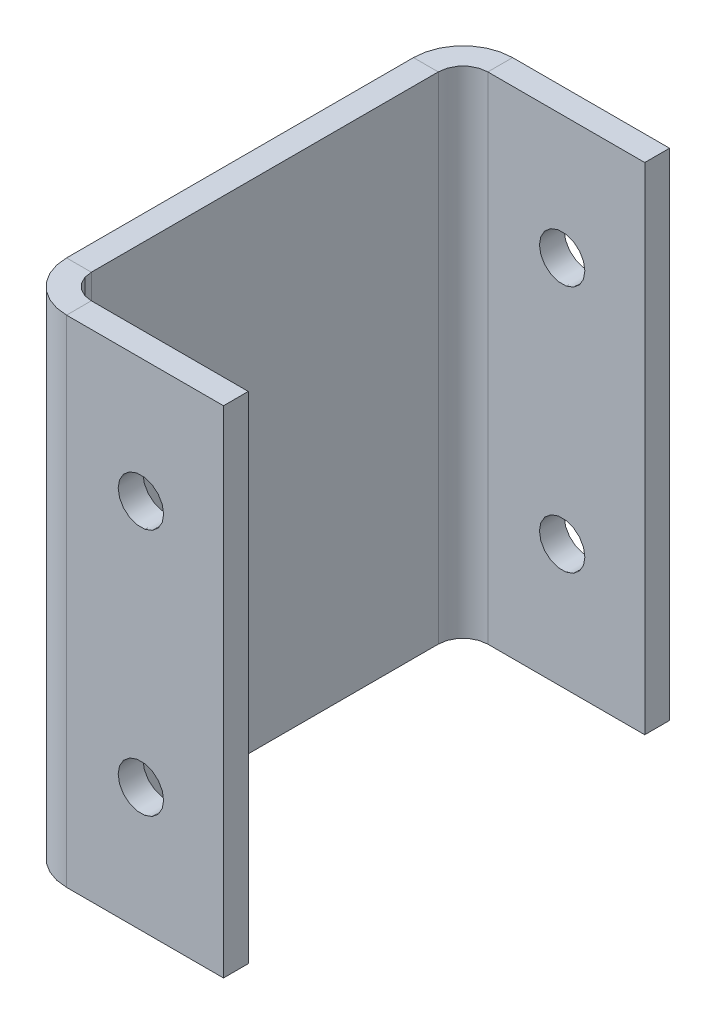
# Autodesk Inventor part: Frontal Sheet Metal Support
Saved by Autodesk Inventor 2019.4 (Build 234330000, 330)
## iProperties
Created: 2020-01-05
Part Number: Frontal Sheet Metal Support
Material: Aluminum 6061
Document SubType Name: Sheet Metal
Designer: Mark
Density: 2.7 g/cm^3
Sheet Metal Rule: Default_mm
Appearance: Aluminum - Flat
Author: Mark
Autodesk Inventor part; units mm, degrees
ref_plane "YZ Plane" through (0, 0, 0) normal (1, 0, 0) x (0, 1, 0)
ref_plane "XZ Plane" through (0, 0, 0) normal (0, 1, 0) x (-1, 0, 0)
ref_plane "XY Plane" through (0, 0, 0) normal (0, 0, 1) x (1, 0, 0)
sketch "Sketch1" plane through (0, 0, 0) normal (1, 0, 0) x (0, 1, 0)
  line L0 (-30, 27) -> (30, 27)
  line L1 (30, 27) -> (30, -27)
  line L2 (30, -27) -> (-30, -27)
  line L3 (-30, -27) -> (-30, 27)
  line L4 (-30, 27) -> (30, -27) construction
  line L5 (30, 27) -> (-30, -27) construction
  point P0 (0, 0)
  dimension "d0" = 60
  dimension "d1" = 54
  measures "d0" distance of L1.end L2.end
  measures "d1" distance of L0.end L1.end
extrude "Plate1" add sketch "Sketch1" along normal blind 3
sketch "Sketch2" plane through (0, -30, 24) normal (0, 0, 1) x (1, 0, 0)
  line L0 (0, 60) -> (0, 0)
  line L1 (0, 0) -> (25, 0)
  line L2 (25, 0) -> (25, 60)
  line L3 (25, 60) -> (0, 60)
  constraints: 6 end point, 1 horizontal, 1 perpendicular, 1 vertical
edge flange "Flange1" height 25 angle 90 thickness 3 bend radius 3 thickness toward (0, 0, 1) relief straight relief width 3 relief depth 1.5 corner gap 3 corner form 0 edges at (3, 0, 27) (3, 0, -27) wall of the first edge with corners at (0, 30, 24) (0, -30, 24) (25, -30, 24) (25, 30, 24)
bend "Bend1"
corner "Corner1"
sketch "Sketch3" plane through (25, -30, 27) normal (0, 0, 1) x (1, 0, 0)
  circle A0 centre (-10, 15) radius 2.75
  circle A1 centre (-10, 45) radius 2.75
  line L0 (0, 0) -> (-19, 0) projected
  line L1 (0, 60) -> (0, 0) projected
  point P0 (-25, 30)
  dimension "d13" = 5.5
  dimension "d14" = 5.5
  dimension "d15" = 30
  dimension "d16" = 15
  dimension "d17" = 10
  dimension "d18" = 10
  constraints: 2 centre point
  measures "d13" diameter of A0
  measures "d14" diameter of A1
  measures "d15" distance of A0.centre A1.centre
  measures "d16" distance from line of L0 A0.centre
  measures "d17" distance from line of L1 A0.centre
  measures "d18" distance from line of L1 A1.centre
extrude "Extrusion1" cut sketch "Sketch3" against normal up to surface (54 mm away)
equation "\"d2\" = Thickness"
equation "\"d3\" = BendReliefWidth"
equation "\"d4\" = BendReliefDepth"
equation "\"d5\" = MinimumRemnant"
equation "\"d6\" = TransitionRadius"
equation "\"d9\" = BendRadius"
equation "\"d10\" = CornerReliefSize"
equation "\"d11\" = GapSize"
equation "\"d12\" = JacobiRadiusSize"
equation "\"BendRadius\" = Thickness"
equation "\"BendReliefWidth\" = Thickness"
equation "\"BendReliefDepth\" = 0.5 * Thickness"
equation "\"CornerReliefSize\" = 4 * Thickness"
equation "\"MinimumRemnant\" = 2 * Thickness"
equation "\"TransitionRadius\" = BendRadius"
equation "\"JacobiRadiusSize\" = BendRadius"
equation "\"GapSize\" = Thickness"
equation "\"Thickness\" = 3"
body "Solid1"
